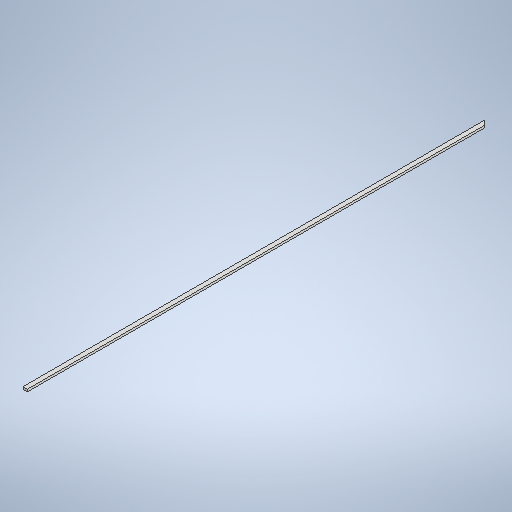
# Autodesk Inventor part: Dichtung_Rechts
Saved by Autodesk Inventor 2025.1 (Build 291241000, 241)
## iProperties
Created: 2024-08-07
Part Number: Dichtung_Rechts
Material: Generisch
Document SubType Name: Modeling
Designer: ffogue
Density: 1 g/cm^3
Appearance: Vorgabe
Author: ffogue
Autodesk Inventor part; units mm, degrees
ref_plane "YZ Plane" through (0, 0, 0) normal (1, 0, 0) x (0, 1, 0)
ref_plane "XZ Plane" through (0, 0, 0) normal (0, 1, 0) x (-1, 0, 0)
ref_plane "XY Plane" through (0, 0, 0) normal (0, 0, 1) x (1, 0, 0)
sketch "Sketch1" plane through (0, 0, 0) normal (0, 0, 1) x (1, 0, 0)
  line L0 (0, 0) -> (19, 0)
  line L1 (19, 0) -> (19, 2000)
  line L2 (19, 2000) -> (0, 2000)
  line L3 (0, 2000) -> (0, 0)
  dimension "d0" = 19
  dimension "d1" = 2000
  constraints: 8 end point, 3 perpendicular, 1 horizontal
  measures "d0" distance between parallel lines of L1 L3
  measures "d1" distance of L2.end L0.start
extrude "Extrusion1" add sketch "Sketch1" along normal blind 10
sketch "Sketch2" plane through (0, 0, 10) normal (0, 0, 1) x (1, 0, 0)
  line L0 (19, 0) -> (19, 2000) projected
  line L1 (19, 2000) -> (0, 2000) projected
  line L2 (0, 2000) -> (0, 0) projected
  line L3 (0, 0) -> (19, 0) projected
  line L4 (0, 2000) -> (19, 1981)
  dimension "d7" = 45
  constraints: 2 end point, 1 point on line
  measures "d7" angle of L1 L4
extrude "Extrusion2" cut sketch "Sketch2" against normal blind 10 contours L4 L1 L0
sketch "Sketch3" plane through (0, 0, 10) normal (0, 0, 1) x (1, 0, 0)
  circle A0 centre (9.5, 210) radius 3
  circle A1 centre (9.5, 170) radius 3
  line L0 (0, 0) -> (19, 0) projected
  point P0 (9.5, 0)
  dimension "d8" = 6
  dimension "d9" = 40
  dimension "d10" = 170
  constraints: 2 centre point, 2 vertical alignment, 1 equal radius, 1 midpoint
  measures "d8" diameter of A0
  measures "d9" distance of A1.centre A0.centre
  measures "d10" distance from line of L0 A1.centre
body "Solid1"
